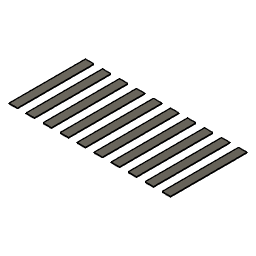
Weave (Autodesk Fusion 360 design; units mm, degrees)
Autodesk Fusion 360 part; units mm, degrees
sketch "Sketch1" plane through (0, 0, 0) normal (0, 0, 1) x (1, 0, 0)
  line L0 (0, 0) -> (10, 0)
  line L1 (10, 0) -> (10, 90)
  line L2 (10, 90) -> (0, 90)
  line L3 (0, 90) -> (0, 0)
  line L4 (20, 90) -> (20, 0)
  line L5 (30, 0) -> (30, 90)
  line L6 (20, 0) -> (30, 0)
  line L7 (30, 90) -> (20, 90)
  line L8 (40, 90) -> (40, 0)
  line L9 (50, 0) -> (50, 90)
  line L10 (40, 0) -> (50, 0)
  line L11 (50, 90) -> (40, 90)
  line L12 (60, 90) -> (60, 0)
  line L13 (70, 0) -> (70, 90)
  line L14 (60, 0) -> (70, 0)
  line L15 (70, 90) -> (60, 90)
  line L16 (80, 90) -> (80, 0)
  line L17 (90, 0) -> (90, 90)
  line L18 (80, 0) -> (90, 0)
  line L19 (90, 90) -> (80, 90)
  line L20 (100, 90) -> (100, 0)
  line L21 (110, 0) -> (110, 90)
  line L22 (100, 0) -> (110, 0)
  line L23 (110, 90) -> (100, 90)
  line L24 (120, 90) -> (120, 0)
  line L25 (130, 0) -> (130, 90)
  line L26 (120, 0) -> (130, 0)
  line L27 (130, 90) -> (120, 90)
  line L28 (140, 90) -> (140, 0)
  line L29 (150, 0) -> (150, 90)
  line L30 (140, 0) -> (150, 0)
  line L31 (150, 90) -> (140, 90)
  line L32 (160, 90) -> (160, 0)
  line L33 (170, 0) -> (170, 90)
  line L34 (160, 0) -> (170, 0)
  line L35 (170, 90) -> (160, 90)
  line L36 (180, 90) -> (180, 0)
  line L37 (190, 0) -> (190, 90)
  line L38 (180, 0) -> (190, 0)
  line L39 (190, 90) -> (180, 90)
  point P0 (20, 0)
  point P1 (40, 0)
  point P2 (60, 0)
  point P3 (80, 0)
  point P4 (100, 0)
  point P5 (120, 0)
  point P6 (140, 0)
  point P7 (160, 0)
  point P8 (180, 0)
  dimension "d1" = 10
  dimension "d2" = 90
  dimension "d5" = 20
  dimension "d6" = 0
  constraint horizontal L0
  constraint vertical L1
  constraint horizontal L2
  constraint vertical L3
  constraint coincident L0.start L3.end
  measures "d1" distance of L0.start L0.end
  measures "d2" distance of L0.start L2.end
extrude "Extrude1" add sketch "Sketch1" along normal blind 0.5 makes body 1 at (63.3333, 60, 0) makes body 2 at (23.3333, 60, 0) makes body 3 at (3.3333, 60, 0) makes body 4 at (123.3333, 60, 0) makes body 5 at (143.3333, 60, 0) makes body 6 at (83.3333, 60, 0) makes body 7 at (183.3333, 60, 0) makes body 8 at (163.3333, 60, 0) makes body 9 at (103.3333, 60, 0) makes body 10 at (43.3333, 60, 0)
